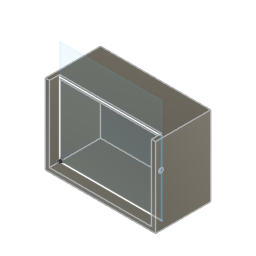
battery_lid (Autodesk Fusion 360 design; units mm, degrees)
Autodesk Fusion 360 part; units mm, degrees
sketch "Sketch3" plane through (0, 106, 0) normal (0, 1, 0) x (-1, 0, 0)
  line L0 (0, -36) -> (0, 15)
  line L1 (0, 15) -> (-50, 15)
  line L2 (-50, 15) -> (-50, -36)
  line L3 (-50, -36) -> (0, -36)
  line L4 (0, -36) -> (-50, -36)
  line L5 (-50, -36) -> (-50, 0)
  line L6 (-50, 0) -> (0, 0)
  line L7 (0, 0) -> (0, -36)
  dimension "d1" = 36
  constraint horizontal L4
  constraint vertical L5
  constraint horizontal L6
  constraint vertical L7
  constraint coincident L0.start L3.end
  measures "d1" distance of L0.start L6.end
sketch "Sketch1" plane through (0, 106, 0) normal (0, 1, 0) x (-1, 0, 0)
  line L0 (-50, 1) -> (0, 1)
  line L1 (0, 1) -> (0, -36)
  line L2 (0, -36) -> (-50, -36)
  line L3 (-50, -36) -> (-50, 1)
  constraint horizontal L0
  constraint vertical L1
  constraint horizontal L2
  constraint vertical L3
extrude "Extrude1" add sketch "Sketch1" along normal blind 22
extrude "Extrude2" add 1 faces at (50, 113.3333, -23.6667) along direction (1, 0, 0) blind 2
extrude "Extrude3" add 1 faces at (0, 113.3333, -11.3333) along direction (-1, 0, 0) blind 2
extrude "Extrude4" add 1 faces at (16, 113.3333, -36) along direction (0, 0, -1) blind 2
extrude "Extrude5" add 1 faces at (34, 106, -25) along direction (0, -1, 0) blind 5
shell "Shell1" thickness 2 removed faces 1 at (34, 101, -25)
sketch "Sketch2" plane through (0, 101, 0) normal (0, -1, 0) x (1, 0, 0)
  line L0 (50, -36) -> (0, -36)
  line L1 (0, -36) -> (0, -1)
  line L2 (0, -1) -> (50, -1)
  line L3 (50, -1) -> (50, -36)
  line L4 (52, -38) -> (52, 1)
  line L5 (52, 1) -> (-2, 1)
  line L6 (-2, 1) -> (-2, -38)
  line L7 (-2, -38) -> (52, -38)
  line L8 (0, 1) -> (50, 1)
  line L9 (50, 1) -> (50, -1)
  line L10 (50, -1) -> (0, -1)
  line L11 (0, -1) -> (0, 1)
  constraint horizontal L8
  constraint vertical L9
  constraint horizontal L10
  constraint vertical L11
  constraint coincident L2.end L3.start
  constraint coincident L5 L8.start
extrude "Extrude6" cut sketch "Sketch2" against normal blind 5 contours L2 L5 L8 L9 L10 L11
hole "Hole1" at (52, 103.6557, -12.4599) direction (-1, 0, 0) diameter 1.623 depth 26 tip angle 118 counterbore diameter 2.2 counterbore depth 1
thread "Thread1" "ISO Metric profile 2.0 M2x0.4 6H" major diameter 2.074 minor diameter 1.623 pitch 0.4 angle 60 modelled right hand crest width 0.1065 on face at (50.6667, 103.3405, -13.2076) crest through (50.9, 104.4672, -12.4599)
ref_plane "WorkPlane1" through (25, 114.5, -18.5) normal (1, 0, 0) x (0, 0, -1)
hole "Hole2" [suppressed]
thread "Thread2" [no effect]
hole "Hole3" [suppressed]
thread "Thread3" [no effect]
